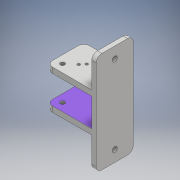
# Autodesk Inventor part: Czesc_do_Ramy
Saved by Autodesk Inventor 2017 (Build 210142000, 142)
## iProperties
Created: 2019-10-29
Part Number: Czesc_do_Ramy
Material: Ogólny
Document SubType Name: Modeling
Designer: patry
Density: 1 g/cm^3
Appearance: Domyślna
Author: patry
Autodesk Inventor part; units mm, degrees
ref_plane "YZ Plane" through (0, 0, 0) normal (1, 0, 0) x (0, 1, 0)
ref_plane "XZ Plane" through (0, 0, 0) normal (0, 1, 0) x (-1, 0, 0)
ref_plane "XY Plane" through (0, 0, 0) normal (0, 0, 1) x (1, 0, 0)
sketch "Szkic1" plane through (0, 0, 0) normal (0, 0, 1) x (1, 0, 0)
  circle A0 centre (0, 0) radius 55 construction
  circle A1 centre (137.9996, 0.347) radius 55 construction
  circle A2 centre (275.9991, 0.6941) radius 55 construction
  line L0 (-173.3991, 195.8773) -> (-173.4121, 201.0636) construction
  line L1 (-173.3991, 247) -> (-173.3991, -116) construction
  line L2 (275.9991, -54.3059) -> (-673, -54.3059) construction
  line L3 (-488.3991, -4.3059) -> (-438.3991, -4.3059) construction
  line L4 (-438.3991, -4.3059) -> (-438.3991, -54.3059) construction
  line L5 (-438.3991, -54.3059) -> (-488.3991, -54.3059) construction
  line L6 (-488.3991, -54.3059) -> (-488.3991, -4.3059) construction
  line L7 (-438.4326, 222.6941) -> (233, 222.6941) construction
  line L8 (-438.4326, 192.6941) -> (378, 192.6941) construction
  line L9 (-476, 207.6941) -> (256, 207.6941) construction
  line L10 (-173.3991, 192.6941) -> (-177.3991, 192.6941)
  line L11 (-177.3991, 192.6941) -> (-177.3991, 225.6941)
  line L12 (-177.3991, 225.6941) -> (-173.3991, 225.6941)
  line L13 (-173.3991, 225.6941) -> (-173.3991, 192.6941)
  point P0 (15, -3)
  dimension "d0" = 50
  dimension "d1" = 50
  dimension "d2" = 265
  dimension "d3" = 277
  dimension "d4" = 30
  dimension "d5" = 15
  dimension "d6" = 4
  dimension "d62" = 33
  constraints: 28 end point, 6 horizontal, 6 parallel, 3 point on line, 2 centre point, 2 perpendicular, 2 vertical, 1 vertical alignment, 2 other
  measures "d0" distance of L4.end L5.end
  measures "d1" distance of L3.end L4.end
  measures "d2" distance between parallel lines of L1 L4
  measures "d3" distance between parallel lines of L2 L7
  measures "d4" distance between parallel lines of L7 L8
  measures "d5" distance between parallel lines of L7 L9
  measures "d6" distance of L11.end L12.end
  measures "d62" distance of L12.end L10.start
extrude "Wyciągnięcie proste1" add sketch "Szkic1" along normal blind 90
sketch "Szkic2" plane through (-177.3991, 192.6941, 0) normal (-1, 0, 0) x (0, 0, 1)
  line L0 (90, 0) -> (90, 33) projected
  line L1 (0, 0) -> (0, 33) projected
  line L2 (0, 0) -> (0, 33) projected
  line L3 (0, 0) -> (90, 0) projected
  line L4 (90, 33) -> (90, 0) projected
  line L5 (0, 33) -> (90, 33) projected
  line L6 (0, 33) -> (90, 33) projected
  line L7 (0, 0) -> (90, 0) projected
  line L8 (57.5, 33) -> (62.5, 33)
  line L9 (62.5, 33) -> (62.5, 0)
  line L10 (62.5, 0) -> (57.5, 0)
  line L11 (57.5, 0) -> (57.5, 33)
  line L12 (32.5, 33) -> (27.5, 33)
  line L13 (27.5, 33) -> (27.5, 0)
  line L14 (27.5, 0) -> (32.5, 0)
  line L15 (32.5, 0) -> (32.5, 33)
  point P0 (0, -192.6941)
  point P1 (80, 16)
  point P2 (10, 16)
  dimension "d9" = 10
  dimension "d10" = 10
  dimension "d11" = 5
  dimension "d12" = 5
  dimension "d13" = 17.5
  dimension "d14" = 17.5
  constraints: 16 end point, 4 parallel, 4 point on line, 2 horizontal, 2 perpendicular
  measures "d9" distance from line of L0 point (80, 16)
  measures "d10" distance from line of L1 point (10, 16)
  measures "d11" distance of L9.end L10.end
  measures "d12" distance of L14.end L13.end
  measures "d13" distance from line of point (80, 16) L9
  measures "d14" distance from line of point (10, 16) L13
extrude "Wyciągnięcie proste2" add sketch "Szkic2" along normal blind 40 contours L3 L11 L5 L9 | L3 L13 L5 L15
fillet "Zaokrąglenie1" radius 5 8 edges at (-217.3991, 192.6941, 60) (-217.3991, 225.6941, 60) (-217.3991, 225.6941, 30) (-217.3991, 192.6941, 30) (-175.3991, 192.6941, 90) (-175.3991, 225.6941, 90) (-175.3991, 225.6941, 0) (-175.3991, 192.6941, 0)
sketch "Szkic3" plane through (-177.3991, 192.6941, 62.5) normal (0, 0, 1) x (1, 0, 0)
  line L0 (-298.6009, 15) -> (433.3991, 15) construction
  line L1 (-40, 5) -> (-40, 28) projected
  line L2 (-311, -197) -> (-261, -197) construction
  line L3 (-261, -247) -> (-311, -247) construction
  line L4 (-497, -197) -> (104, -197) construction
  line L5 (-221, 86) -> (-221, -341.1695) construction
  line L6 (-246, 90.4419) -> (-246, -336.7276) construction
  line L7 (-296, 88) -> (-296, -339.1695) construction
  line L8 (-271, 89) -> (-271, -338.1695) construction
  line L9 (4, 54.3059) -> (4, -308.6941) construction
  line L10 (-221, -197) -> (144.5683, 199.6805) construction
  line L11 (-246, -197) -> (156.8943, 188.8706) construction
  line L12 (-271, -197) -> (64.3345, 90.4296) construction
  line L13 (-296, -197) -> (182.0787, 173.8291) construction
  line L14 (-196, -338.1695) -> (-196, 81) construction
  line L15 (-171, -340.9749) -> (-171, 78.1946) construction
  line L16 (-296, -333) -> (-296, 85.2632) construction
  line L17 (-321, 80.9017) -> (-321, -346.2678) construction
  line L18 (-196, -197) -> (27.7781, 83.0658) construction
  circle A0 centre (-33, 7) radius 26.5 construction
  circle A1 centre (-33, 7) radius 24 construction
  circle A2 centre (-33, 7) radius 19 construction
  circle A3 centre (-33, 7) radius 25.25 construction
  circle A4 centre (-33, 7) radius 21.5 construction
  circle A5 centre (-33, 7) radius 20.25 construction
  circle A6 centre (-33, 7) radius 31.5 construction
  circle A7 centre (-33, 7) radius 16.5 construction
  circle A8 centre (-33, 7) radius 15.25 construction
  circle A9 centre (-33, 7) radius 14 construction
  circle A10 centre (-33, 7) radius 11.5 construction
  circle A11 centre (-33, 7) radius 10.25 construction
  circle A12 centre (-33, 7) radius 9 construction
  point P0 (177.3991, -192.6941)
  point P1 (-33, 15)
  point P2 (-13.0484, 22.4757)
  point P3 (-21.9865, 17.5482)
  point P4 (-25.2176, 13.6706)
  point P5 (-19.277, 21.891)
  point P6 (-17.2382, 26.7264)
  dimension "d33" = 40.5
  dimension "d36" = 30.5
  dimension "d46" = 20.5
  dimension "d18" = 7
  dimension "d19" = 8
  dimension "d20" = 225
  dimension "d21" = 250
  dimension "d22" = 275
  dimension "d24" = 200
  dimension "d25" = 175
  dimension "d26" = 300
  dimension "d27" = 325
  dimension "d28" = 53
  dimension "d29" = 48
  dimension "d30" = 38
  dimension "d31" = 50.5
  dimension "d32" = 43
  dimension "d34" = 63
  dimension "d35" = 33
  dimension "d37" = 28
  dimension "d45" = 23
  dimension "d47" = 18
  constraints: 28 end point, 22 point on line, 13 coincident, 10 centre point, 8 vertical, 2 point on circle, 1 horizontal, 1 vertical alignment, 9 other
  measures "d18" distance from line of L1 point (-33, 15)
  measures "d19" distance of point (-33, 15) point (-33, 7)
  measures "d20" distance from line of L9.end L5
  measures "d21" distance between parallel lines of L9 L6
  measures "d22" distance between parallel lines of L9 L8
  measures "d24" distance between parallel lines of L9 L14
  measures "d25" distance between parallel lines of L9 L15
  measures "d26" distance from line of L9.end L16
  measures "d27" distance from line of L9 L17.end
  measures "d28" diameter of A0
  measures "d29" diameter of A1
  measures "d30" diameter of A2
  measures "d31" diameter of A3
  measures "d32" diameter of A4
  measures "d34" diameter of A6
  measures "d35" diameter of A7
  measures "d37" diameter of A9
  measures "d45" diameter of A10
  measures "d47" diameter of A12
hole "Otwór2" at (-190.4475, 215.1698, 62.5) at (-199.3855, 210.2423, 62.5) at (-202.6167, 206.3647, 62.5) at (-196.676, 214.585, 62.5) at (-194.6373, 219.4204, 62.5) direction (0, 0, -1) diameter 2.4 depth 8 tip angle 118 clearance for "Śruba ze łbem płaskim obrobiona" size "M2" standard "ANSI Profil metryczny M"
hole "Otwór3" at (-210.3991, 199.6941, 62.5) direction (0, 0, -1) diameter 3.9 end through all clearance for "Śruba ze łbem płaskim obrobiona" size "M3.5" standard "ANSI Profil metryczny M"
sketch "Szkic4" plane through (-173.3991, 197.6941, 0) normal (1, 0, 0) x (0, 0, -1)
  line L0 (-90, 23) -> (-90, 0) projected
  line L1 (-5, 28) -> (-85, 28) projected
  point P0 (0, -197.6941)
  point P1 (-80, 11.5)
  point P2 (-10, 11.5)
  dimension "d63" = 70
  dimension "d64" = 10
  dimension "d65" = 16.5
  constraints: 1 horizontal alignment
  measures "d63" distance of point (-10, 11.5) point (-80, 11.5)
  measures "d64" distance from line of L0 point (-80, 11.5)
  measures "d65" distance from line of point (-80, 11.5) L1
hole "Otwór4" at (-173.3991, 209.1941, 80) at (-173.3991, 209.1941, 10) direction (-1, 0, 0) diameter 4.5 depth 8 tip angle 118 clearance for "Śruba ze łbem płaskim obrobiona" size "M4" standard "ANSI Profil metryczny M"
equation "\"d5\" = 0.5 * d4"
equation "\"d9\" = d10"
equation "\"d14\" = d13"
